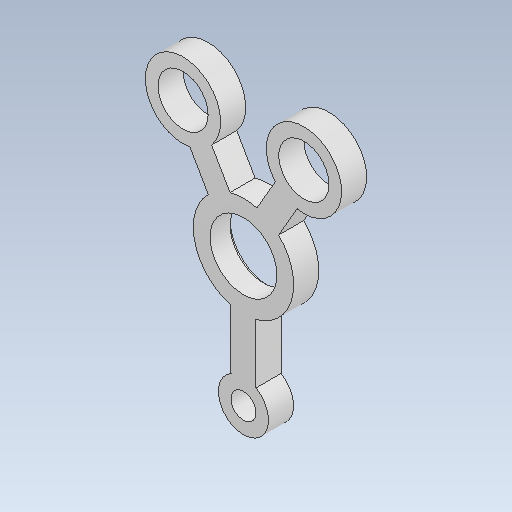
# Autodesk Inventor part: 中間ギア抑え
Saved by Autodesk Inventor 2020.2 (Build 242310000, 310)
## iProperties
Created: 2020-03-12
Part Number: 中間ギア抑え
Material: アルミニウム 2014-T4
Document SubType Name: Modeling
Designer: aoyam
Density: 2.8 g/cm^3
Appearance: サテン
Mass: 1.64798 g
Surface Area: 9.97527 cm^2
Volume: 0.588564 cm^3
Author: aoyam
Autodesk Inventor part; units mm, degrees
ref_plane "YZ Plane" through (0, 0, 0) normal (1, 0, 0) x (0, 1, 0)
ref_plane "XZ Plane" through (0, 0, 0) normal (0, 1, 0) x (-1, 0, 0)
ref_plane "XY Plane" through (0, 0, 0) normal (0, 0, 1) x (1, 0, 0)
sketch "スケッチ1" plane through (0, 0, 0) normal (0, 0, 1) x (1, 0, 0)
  circle A0 centre (0, 15.5) radius 3 construction
  circle A1 centre (0, -15.5) radius 1.5
  circle A2 centre (0, 15.5) radius 4.5 construction
  circle A3 centre (0, -15.5) radius 3
  line L0 (0, 15.5) -> (0, -15.5) construction
  line L1 (-1.5, 15.5) -> (-1.5, -15.5)
  line L2 (1.5, -15.5) -> (1.5, 15.5)
  arc A4 (1.5, 15.5) -> (-1.5, 15.5) centre (0, 15.5) ccw
  arc A5 (-1.5, -15.5) -> (1.5, -15.5) centre (0, -15.5) ccw
  circle A6 centre (0, 0) radius 6
  circle A7 centre (0, 0) radius 4
  circle A8 centre (0, 0) radius 4.6
  line L3 (0, 0) -> (-7.2283, 12.5198) construction
  line L4 (1.299, 0.75) -> (-5.9293, 13.2698)
  line L5 (-8.5273, 11.7698) -> (-1.299, -0.75)
  arc A9 (-1.299, -0.75) -> (1.299, 0.75) centre (0, 0) ccw
  arc A10 (-5.9293, 13.2698) -> (-8.5273, 11.7698) centre (-7.2283, 12.5198) ccw
  circle A11 centre (-7.2283, 12.5198) radius 3
  circle A12 centre (0, 15.5) radius 3 construction
  circle A13 centre (0, 15.5) radius 4.5 construction
  line L6 (-1.299, 0.75) -> (5.9293, 13.2698)
  line L7 (8.5273, 11.7698) -> (1.299, -0.75)
  circle A14 centre (7.2283, 12.5198) radius 3
  circle A15 centre (-7.2283, 12.5198) radius 1.5
  circle A16 centre (7.2283, 12.5198) radius 1.5
  circle A17 centre (-7.2283, 12.5198) radius 4.5
  circle A18 centre (7.2283, 12.5198) radius 4.5
  point P0 (0, 0)
  point P1 (0, 0)
  point P2 (-1.5, 11.2574)
  point P3 (-1.5, 5.8095)
  point P4 (-1.5, -5.8095)
  point P5 (-1.5, -12.9019)
  point P6 (1.5, -12.9019)
  point P7 (1.5, -5.8095)
  point P8 (1.5, 5.8095)
  point P9 (1.5, 11.2574)
  point P10 (-3.6142, 6.2599)
  point P11 (4.2038, 4.2812)
  point P12 (7.2283, 9.5198)
  point P13 (4.6302, 11.0198)
  point P14 (1.6057, 5.7812)
  point P15 (-1.6057, 5.7812)
  point P16 (-4.6302, 11.0198)
  point P17 (-7.2283, 9.5198)
  point P18 (-4.2038, 4.2812)
  point P19 (6.406, 8.0955)
  point P20 (3.8079, 9.5955)
  point P21 (-3.8079, 9.5955)
  point P22 (-6.406, 8.0955)
  dimension "d0" = 12
  dimension "d1" = 8
  dimension "d2" = 9.2
  dimension "d7" = 6
  dimension "d8" = 3
  dimension "d9" = 3
  dimension "d10" = 3
  dimension "d11" = 6
  dimension "d12" = 3
  dimension "d13" = 3
  dimension "d14" = 30
  dimension "d15" = 6
  dimension "d16" = 9
  dimension "d17" = 9
  constraints: 20 end point, 19 centre point, 8 point on circle, 8 tangent, 7 coincident, 6 symmetric about line, 2 midpoint, 2 parallel, 1 point on line, 1 vertical, 3 other
  measures "d0" diameter of A6
  measures "d1" diameter of A7
  measures "d2" diameter of A8
  measures "d7" diameter of A0
  measures "d8" diameter of A1
  measures "d9" distance between parallel lines of L1 L2
  measures "d10" diameter of A10
  measures "d11" diameter of A11
  measures "d12" diameter of A15
  measures "d13" diameter of A16
  measures "d14" angle of L0 L3
  measures "d15" diameter of A3
  measures "d16" diameter of A17
  measures "d17" diameter of A18
extrude "押し出し1" add sketch "スケッチ1" along normal blind 3 contours L2 A3 L1 A1 | A1 L1 A3 L2 | A3 L1 A6 L2 | A6 L1 A8 L2 | L2 A8 L7 A6 | A6 L5 A8 L1 | A8 L1 A7 L2 | L2 A7 L7 A8 | A8 L5 A7 L1 | L5 A17 L4 A6 | A6 L4 L1 A8 L5 | L7 A8 L2 L6 A6 | A6 L6 A18 L7 | A8 L1 A7 L5 | A6 L1 L4 | A17 L4 A11 L5 | L5 A11 L4 A17 | L7 A7 L2 A8 | L6 L2 A6 | A18 L6 A14 L7 | L7 A14 L6 A18 | A8 L4 A7 L1 | L1 L4 A8 | A6 L2 L6 A8 L4 L1 | A8 L6 L2 | L2 A7 L6 A8 | A8 L6 A7 L4
extrude "押し出し2" cut sketch "スケッチ1" along normal blind 0.6 contours A8 L1 A7 L2 | L2 A7 L7 A8 | A8 L5 A7 L1 | A8 L1 A7 L5 | L7 A7 L2 A8 | A8 L4 A7 L1 | L2 A7 L6 A8 | A8 L6 A7 L4
sketch "スケッチ2" plane through (0, 0, 3) normal (0, 0, 1) x (1, 0, 0)
  arc A0 (1.6057, 5.7812) -> (-1.6057, 5.7812) centre (0, 0) ccw projected
  line L0 (-1.5, -5.8095) -> (-1.5, -12.9019) projected
  arc A1 (-1.5, -12.9019) -> (1.5, -12.9019) centre (0, -15.5) ccw projected
  line L1 (1.5, -12.9019) -> (1.5, -5.8095) projected
  arc A2 (1.5, -5.8095) -> (4.2038, 4.2812) centre (0, 0) ccw projected
  circle A3 centre (0, -15.5) radius 1.5 projected
  circle A4 centre (0, 0) radius 4 projected
  arc A5 (-4.2038, 4.2812) -> (-1.5, -5.8095) centre (0, 0) ccw projected
  line L2 (4.2038, 4.2812) -> (6.406, 8.0955) projected
  circle A6 centre (7.2283, 12.5198) radius 3 projected
  line L3 (3.8079, 9.5955) -> (1.6057, 5.7812) projected
  line L4 (-1.6057, 5.7812) -> (-3.8079, 9.5955) projected
  circle A7 centre (-7.2283, 12.5198) radius 3 projected
  line L5 (-6.406, 8.0955) -> (-4.2038, 4.2812) projected
  arc A8 (6.406, 8.0955) -> (3.8079, 9.5955) centre (7.2283, 12.5198) ccw projected
  arc A9 (-3.8079, 9.5955) -> (-6.406, 8.0955) centre (-7.2283, 12.5198) ccw projected
  point P0 (0, 0)
